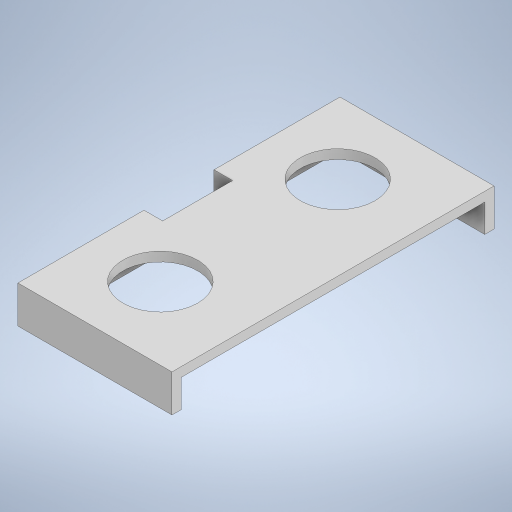
# Autodesk Inventor part: top
Saved by Autodesk Inventor 2023 (Build 270158000, 158)
## iProperties
Created: 2023-05-02
Part Number: top
Material: Generic
Document SubType Name: Modeling
Designer: ringl
Density: 1 g/cm^3
Appearance: Default
Author: ringl
Autodesk Inventor part; units mm, degrees
ref_plane "YZ Plane" through (0, 0, 0) normal (1, 0, 0) x (0, 1, 0)
ref_plane "XZ Plane" through (0, 0, 0) normal (0, 1, 0) x (-1, 0, 0)
ref_plane "XY Plane" through (0, 0, 0) normal (0, 0, 1) x (1, 0, 0)
sketch "Sketch1" plane through (0, 0, 0) normal (0, 1, 0) x (-1, 0, 0)
  line L0 (0, 0) -> (33, 0)
  line L1 (33, 0) -> (33, -69)
  line L2 (33, -69) -> (0, -69)
  line L3 (2, -2) -> (31, -2)
  line L4 (31, -2) -> (31, -67)
  line L5 (31, -67) -> (2, -67)
  line L6 (2, -2) -> (0, -2)
  line L7 (2, -67) -> (0, -67)
  line L8 (0, -69) -> (0, -67)
  line L9 (0, -2) -> (0, 0)
  dimension "d0" = 2
  dimension "d1" = 2
  dimension "d3" = 2
  dimension "d4" = 33
  dimension "d5" = 69
  dimension "d7" = 0
  constraints: 20 end point, 6 perpendicular, 4 parallel, 2 horizontal
  measures "d0" distance between parallel lines of L2 L5
  measures "d1" distance between parallel lines of L1 L4
  measures "d3" distance between parallel lines of L0 L3
  measures "d4" distance of L1.end L2.end
  measures "d5" distance of L0.end L1.end
  measures "d7" distance between parallel lines of L9 L8
extrude "Extrusion1" add sketch "Sketch1" along normal blind 6
sketch "Sketch2" plane through (0, 6, 0) normal (0, 1, 0) x (1, 0, 0)
  line L0 (0, 0) -> (0, 2) projected
  line L1 (0, 69) -> (-33, 69) projected
  line L2 (0, 0) -> (-33, 0)
  line L3 (-33, 0) -> (-33, 69)
  line L4 (-33, 69) -> (0, 69)
  line L5 (0, 69) -> (0, 0)
  constraints: 8 end point, 2 parallel, 1 horizontal, 1 perpendicular
extrude "Extrusion2" add sketch "Sketch2" along normal blind 2
sketch "Sketch3" plane through (0, 8, 0) normal (0, 1, 0) x (1, 0, 0)
  circle A0 centre (-18, 15.5) radius 8
  circle A1 centre (-18, 53.5) radius 8
  line L0 (-33, 69) -> (-33, 0) construction
  line L1 (-33, 34.5) -> (0, 34.5) construction
  line L2 (0, 2) -> (0, 67) construction
  line L3 (-33, 0) -> (0, 0) construction
  dimension "d12" = 16
  dimension "d13" = 16
  dimension "d14" = 34.5
  dimension "d15" = 19
  dimension "d16" = 19
  dimension "d17" = 15
  dimension "d18" = 15
  constraints: 2 centre point, 2 end point, 2 midpoint, 1 horizontal
  measures "d12" diameter of A0
  measures "d13" diameter of A1
  measures "d14" distance between parallel lines of L3 L1
  measures "d15" distance from line of A0.centre L1
  measures "d16" distance from line of L1 A1.centre
  measures "d17" distance from line of L0 A1.centre
  measures "d18" distance from line of L0 A0.centre
extrude "Extrusion3" cut sketch "Sketch3" against normal blind 2
sketch "Sketch4" plane through (-33, 0, -69) normal (-1, 0, 0) x (0, 0, 1)
  line L0 (67, 0) -> (2, 0) projected
  line L1 (27, 0) -> (42, 0)
  line L2 (42, 0) -> (42, 8)
  line L3 (42, 8) -> (27, 8)
  line L4 (27, 8) -> (27, 0)
  line L5 (0, 0) -> (0, 8) projected
  point P0 (69, 0)
  dimension "d21" = 15
  dimension "d22" = 27
  dimension "d23" = 8
  constraints: 8 end point, 2 parallel, 1 horizontal, 1 perpendicular, 1 point on line
  measures "d21" distance of L2.end L3.end
  measures "d22" distance between parallel lines of L5 L4
  measures "d23" distance of L1.end L2.end
extrude "Extrusion4" cut sketch "Sketch4" against normal blind 4
body "Solid1"
